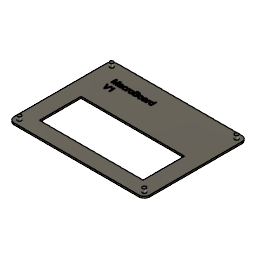
Macro top v1 (Autodesk Fusion 360 design; units mm, degrees)
Autodesk Fusion 360 part; units mm, degrees
sketch "plate-2025-12-30T17_40_52.249Z" plane through (0, 0, 0) normal (0, 0, 1) x (1, 0, 0)
  line L0 (3.025, -2.525) -> (16.025, -2.525)
  line L1 (3.025, -16.525) -> (16.025, -16.525)
  line L2 (2.525, -3.025) -> (2.525, -16.025)
  line L3 (16.525, -3.025) -> (16.525, -16.025)
  arc A0 (3.025, -2.525) -> (2.525, -3.025) centre (3.025, -3.025) ccw
  arc A1 (16.525, -3.025) -> (16.025, -2.525) centre (16.025, -3.025) ccw
  arc A2 (2.525, -16.025) -> (3.025, -16.525) centre (3.025, -16.025) ccw
  arc A3 (16.025, -16.525) -> (16.525, -16.025) centre (16.025, -16.025) ccw
  line L4 (22.075, -2.525) -> (35.075, -2.525)
  line L5 (22.075, -16.525) -> (35.075, -16.525)
  line L6 (21.575, -3.025) -> (21.575, -16.025)
  line L7 (35.575, -3.025) -> (35.575, -16.025)
  arc A4 (22.075, -2.525) -> (21.575, -3.025) centre (22.075, -3.025) ccw
  arc A5 (35.575, -3.025) -> (35.075, -2.525) centre (35.075, -3.025) ccw
  arc A6 (21.575, -16.025) -> (22.075, -16.525) centre (22.075, -16.025) ccw
  arc A7 (35.075, -16.525) -> (35.575, -16.025) centre (35.075, -16.025) ccw
  line L8 (41.125, -2.525) -> (54.125, -2.525)
  line L9 (41.125, -16.525) -> (54.125, -16.525)
  line L10 (40.625, -3.025) -> (40.625, -16.025)
  line L11 (54.625, -3.025) -> (54.625, -16.025)
  arc A8 (41.125, -2.525) -> (40.625, -3.025) centre (41.125, -3.025) ccw
  arc A9 (54.625, -3.025) -> (54.125, -2.525) centre (54.125, -3.025) ccw
  arc A10 (40.625, -16.025) -> (41.125, -16.525) centre (41.125, -16.025) ccw
  arc A11 (54.125, -16.525) -> (54.625, -16.025) centre (54.125, -16.025) ccw
  line L12 (60.175, -2.525) -> (73.175, -2.525)
  line L13 (60.175, -16.525) -> (73.175, -16.525)
  line L14 (59.675, -3.025) -> (59.675, -16.025)
  line L15 (73.675, -3.025) -> (73.675, -16.025)
  arc A12 (60.175, -2.525) -> (59.675, -3.025) centre (60.175, -3.025) ccw
  arc A13 (73.675, -3.025) -> (73.175, -2.525) centre (73.175, -3.025) ccw
  arc A14 (59.675, -16.025) -> (60.175, -16.525) centre (60.175, -16.025) ccw
  arc A15 (73.175, -16.525) -> (73.675, -16.025) centre (73.175, -16.025) ccw
  line L16 (79.225, -2.525) -> (92.225, -2.525)
  line L17 (79.225, -16.525) -> (92.225, -16.525)
  line L18 (78.725, -3.025) -> (78.725, -16.025)
  line L19 (92.725, -3.025) -> (92.725, -16.025)
  arc A16 (79.225, -2.525) -> (78.725, -3.025) centre (79.225, -3.025) ccw
  arc A17 (92.725, -3.025) -> (92.225, -2.525) centre (92.225, -3.025) ccw
  arc A18 (78.725, -16.025) -> (79.225, -16.525) centre (79.225, -16.025) ccw
  arc A19 (92.225, -16.525) -> (92.725, -16.025) centre (92.225, -16.025) ccw
  line L20 (3.025, -21.575) -> (16.025, -21.575)
  line L21 (3.025, -35.575) -> (16.025, -35.575)
  line L22 (2.525, -22.075) -> (2.525, -35.075)
  line L23 (16.525, -22.075) -> (16.525, -35.075)
  arc A20 (3.025, -21.575) -> (2.525, -22.075) centre (3.025, -22.075) ccw
  arc A21 (16.525, -22.075) -> (16.025, -21.575) centre (16.025, -22.075) ccw
  arc A22 (2.525, -35.075) -> (3.025, -35.575) centre (3.025, -35.075) ccw
  arc A23 (16.025, -35.575) -> (16.525, -35.075) centre (16.025, -35.075) ccw
  line L24 (22.075, -21.575) -> (35.075, -21.575)
  line L25 (22.075, -35.575) -> (35.075, -35.575)
  line L26 (21.575, -22.075) -> (21.575, -35.075)
  line L27 (35.575, -22.075) -> (35.575, -35.075)
  arc A24 (22.075, -21.575) -> (21.575, -22.075) centre (22.075, -22.075) ccw
  arc A25 (35.575, -22.075) -> (35.075, -21.575) centre (35.075, -22.075) ccw
  arc A26 (21.575, -35.075) -> (22.075, -35.575) centre (22.075, -35.075) ccw
  arc A27 (35.075, -35.575) -> (35.575, -35.075) centre (35.075, -35.075) ccw
  line L28 (41.125, -21.575) -> (54.125, -21.575)
  line L29 (41.125, -35.575) -> (54.125, -35.575)
  line L30 (40.625, -22.075) -> (40.625, -35.075)
  line L31 (54.625, -22.075) -> (54.625, -35.075)
  arc A28 (41.125, -21.575) -> (40.625, -22.075) centre (41.125, -22.075) ccw
  arc A29 (54.625, -22.075) -> (54.125, -21.575) centre (54.125, -22.075) ccw
  arc A30 (40.625, -35.075) -> (41.125, -35.575) centre (41.125, -35.075) ccw
  arc A31 (54.125, -35.575) -> (54.625, -35.075) centre (54.125, -35.075) ccw
  line L32 (60.175, -21.575) -> (73.175, -21.575)
  line L33 (60.175, -35.575) -> (73.175, -35.575)
  line L34 (59.675, -22.075) -> (59.675, -35.075)
  line L35 (73.675, -22.075) -> (73.675, -35.075)
  arc A32 (60.175, -21.575) -> (59.675, -22.075) centre (60.175, -22.075) ccw
  arc A33 (73.675, -22.075) -> (73.175, -21.575) centre (73.175, -22.075) ccw
  arc A34 (59.675, -35.075) -> (60.175, -35.575) centre (60.175, -35.075) ccw
  arc A35 (73.175, -35.575) -> (73.675, -35.075) centre (73.175, -35.075) ccw
  line L36 (79.225, -21.575) -> (92.225, -21.575)
  line L37 (79.225, -35.575) -> (92.225, -35.575)
  line L38 (78.725, -22.075) -> (78.725, -35.075)
  line L39 (92.725, -22.075) -> (92.725, -35.075)
  arc A36 (79.225, -21.575) -> (78.725, -22.075) centre (79.225, -22.075) ccw
  arc A37 (92.725, -22.075) -> (92.225, -21.575) centre (92.225, -22.075) ccw
  arc A38 (78.725, -35.075) -> (79.225, -35.575) centre (79.225, -35.075) ccw
  arc A39 (92.225, -35.575) -> (92.725, -35.075) centre (92.225, -35.075) ccw
  line L40 (0, -38.1) -> (95.25, -38.1)
  line L41 (0, 0) -> (95.25, 0)
  line L42 (0, -38.1) -> (0, 0)
  line L43 (95.25, -38.1) -> (95.25, 0)
  line L44 (-14.67, 42.994) -> (110.33, 42.994)
  line L45 (110.33, 42.994) -> (110.33, -52.006)
  line L46 (110.33, -52.006) -> (-14.67, -52.006)
  line L47 (-14.67, -52.006) -> (-14.67, 42.994)
  circle A40 centre (-9.67, 37.994) radius 3
  circle A41 centre (-9.67, 37.994) radius 1.7
  circle A42 centre (105.33, 37.994) radius 1.7
  circle A43 centre (105.33, 37.994) radius 3
  circle A44 centre (105.33, -47.006) radius 3
  circle A45 centre (105.33, -47.006) radius 1.7
  circle A46 centre (-9.67, -47.006) radius 3
  circle A47 centre (-9.67, -47.006) radius 1.7
  dimension "d13" = 125
  dimension "d14" = 95
  dimension "d15" = 13.906
  dimension "d16" = 15.08
  dimension "d17" = 14.67
  dimension "d18" = 6
  dimension "d19" = 5
  dimension "d20" = 5
  dimension "d21" = 3.4
  dimension "d22" = 6
  dimension "d23" = 3.4
  dimension "d24" = 6
  dimension "d25" = 3.4
  dimension "d26" = 6
  dimension "d27" = 3.4
  constraint horizontal L44
  constraint vertical L45
  constraint horizontal L46
  constraint vertical L47
  constraint concentric A40 A41
  constraint concentric A42 A43
  constraint concentric A44 A45
  constraint concentric A46 A47
  measures "d13" distance of L44.start L44.end
  measures "d14" distance of L44.start L46.end
  measures "d15" distance of L40 L46
  measures "d16" distance of L43 L45
  measures "d17" distance of L42 L47
  measures "d18" diameter of A40
  measures "d19" distance of L44 A40.centre
  measures "d20" distance of L47 A40.centre
  measures "d21" diameter of A41
  measures "d22" diameter of A43
  measures "d23" diameter of A42
  measures "d24" diameter of A44
  measures "d25" diameter of A45
  measures "d26" diameter of A46
  measures "d27" diameter of A47
extrude "Extrude1" add sketch "plate-2025-12-30T17_40_52.249Z" along normal blind 1.5 contours L44 L45 L46 L47 | A40 | A43 | A44 | A46
extrude "Extrude2" add sketch "plate-2025-12-30T17_40_52.249Z" along normal blind 5 contours A41 | A42 | A45 | A47
fillet "Fillet1" radius 5 4 edges at (-14.67, -52.006, 0.75) (-14.67, 42.994, 0.75) (110.33, 42.994, 0.75) (110.33, -52.006, 0.75)
sketch "Sketch7" plane through (0, 0, 1.5) normal (0, 0, 1) x (-1, 0, 0)
  circle A0 centre (9.67, -37.994) radius 1.7
  line L0 (-95.25, 38.1) -> (0, 38.1)
  line L1 (0, 38.1) -> (0, 0)
  line L2 (0, 0) -> (-95.25, 0)
  line L3 (-95.25, 0) -> (-95.25, 38.1)
  circle A1 centre (9.67, 47.006) radius 1.7
  circle A2 centre (-105.33, -37.994) radius 1.7
  circle A3 centre (-105.33, 47.006) radius 1.7
  arc A4 (-105.33, 52.006) -> (-110.33, 47.006) centre (-105.33, 47.006) ccw
  line L4 (-110.33, 47.006) -> (-110.33, -37.994)
  arc A5 (-110.33, -37.994) -> (-105.33, -42.994) centre (-105.33, -37.994) ccw
  line L5 (-105.33, -42.994) -> (9.67, -42.994)
  arc A6 (9.67, -42.994) -> (14.67, -37.994) centre (9.67, -37.994) ccw
  line L6 (14.67, -37.994) -> (14.67, 47.006)
  arc A7 (14.67, 47.006) -> (9.67, 52.006) centre (9.67, 47.006) ccw
  line L7 (9.67, 52.006) -> (-105.33, 52.006)
  line L8 (-2, -24) -> (-17, -24) construction
  line L9 (-17, -24) -> (-17, -30) construction
  line L10 (-17, -30) -> (-2, -30) construction
  line L11 (-2, -30) -> (-2, -24) construction
  dimension "d34" = 5
  text T0 "MacroBoard V1\n" font "Arial" height 5 align left top in box 15 x 6 at (-2, -24) x (-1, 0) y (0, -1) spacing 1
extrude "Extrude3" cut sketch "Sketch7" against normal blind 0.3 text T0
equation "d35 = 'MacroBoard V1 '"
